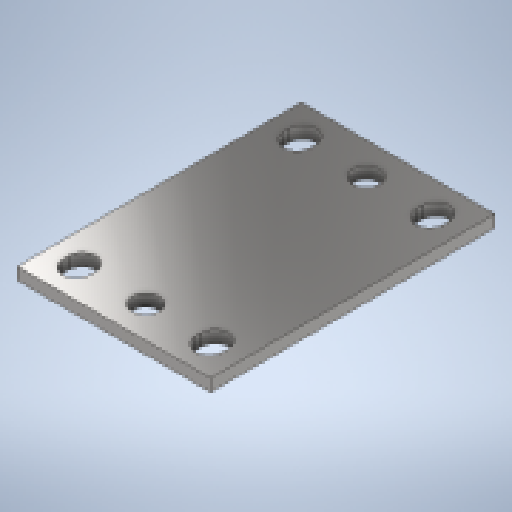
# Autodesk Inventor part: motor_bracket_upper
Saved by Autodesk Inventor 2026.2 (Build 302298010, 298A)
## iProperties
Created: 2026-03-29
Part Number: motor_bracket_upper
Material: Steel, Alloy
Document SubType Name: Modeling
Designer: chanh
Density: 7.73 g/cm^3
Appearance: Semi-Polished
Author: chanh
Autodesk Inventor part; units mm, degrees
ref_plane "YZ Plane" through (0, 0, 0) normal (1, 0, 0) x (0, 1, 0)
ref_plane "XZ Plane" through (0, 0, 0) normal (0, 1, 0) x (-1, 0, 0)
ref_plane "XY Plane" through (0, 0, 0) normal (0, 0, 1) x (1, 0, 0)
sketch "Sketch1" plane through (0, 0, 0) normal (0, 1, 0) x (-1, 0, 0)
  circle A0 centre (0, 0) radius 20
  dimension "d0" = 40
  constraints: 1 centre point, 1 coincident
  measures "d0" diameter of A0
extrude "Extrusion1" add sketch "Sketch1" along normal blind 5
sketch "Sketch2" plane through (0, 5, 0) normal (0, 1, 0) x (1, 0, 0)
  line L0 (-32, -47) -> (32, -47)
  line L1 (32, -47) -> (32, 47)
  line L2 (32, 47) -> (-32, 47)
  line L3 (-32, 47) -> (-32, -47)
  line L4 (-32, -47) -> (32, 47) construction
  line L5 (32, -47) -> (-32, 47) construction
  line L6 (-22, -36.5) -> (22, -36.5) construction
  line L7 (22, -36.5) -> (22, 36.5) construction
  line L8 (22, 36.5) -> (-22, 36.5) construction
  line L9 (-22, 36.5) -> (-22, -36.5) construction
  line L10 (-22, -36.5) -> (22, 36.5) construction
  line L11 (22, -36.5) -> (-22, 36.5) construction
  line L12 (-22, 35.5) -> (-22, 37.5) construction
  line L13 (-17.5, 35.5) -> (-17.5, 37.5)
  line L14 (-26.5, 37.5) -> (-26.5, 35.5)
  arc A0 (-26.5, 35.5) -> (-17.5, 35.5) centre (-22, 35.5) ccw
  arc A1 (-17.5, 37.5) -> (-26.5, 37.5) centre (-22, 37.5) ccw
  line L15 (-32, 0) -> (32, 0) construction
  line L16 (0, 47) -> (0, -47) construction
  line L17 (17.5, 35.5) -> (17.5, 37.5)
  line L18 (26.5, 37.5) -> (26.5, 35.5)
  arc A2 (17.5, 35.5) -> (26.5, 35.5) centre (22, 35.5) ccw
  arc A3 (26.5, 37.5) -> (17.5, 37.5) centre (22, 37.5) ccw
  line L19 (-17.5, -35.5) -> (-17.5, -37.5)
  line L20 (-26.5, -37.5) -> (-26.5, -35.5)
  arc A4 (-17.5, -35.5) -> (-26.5, -35.5) centre (-22, -35.5) ccw
  arc A5 (-26.5, -37.5) -> (-17.5, -37.5) centre (-22, -37.5) ccw
  arc A6 (17.5, -37.5) -> (26.5, -37.5) centre (22, -37.5) ccw
  line L21 (26.5, -37.5) -> (26.5, -35.5)
  arc A7 (26.5, -35.5) -> (17.5, -35.5) centre (22, -35.5) ccw
  line L22 (17.5, -35.5) -> (17.5, -37.5)
  circle A8 centre (0, 36.5) radius 4.5
  circle A9 centre (0, -36.5) radius 4.5
  point P0 (0, 0)
  dimension "d3" = 64
  dimension "d4" = 94
  dimension "d5" = 44
  dimension "d6" = 73
  dimension "d7" = 1
  dimension "d8" = 9
  dimension "d9" = 9
  dimension "d10" = 9
  constraints: 48 end point, 18 symmetric about line, 16 point on circle, 11 midpoint, 10 centre point, 5 parallel, 4 tangent, 3 point on line, 2 horizontal, 2 perpendicular, 6 other
  measures "d3" distance of L1.end L2.end
  measures "d4" distance between parallel lines of L2 L0
  measures "d5" distance of L7.end L8.end
  measures "d6" distance of L6.end L7.end
  measures "d7" distance of L8.end L12.end
  measures "d8" diameter of A1
  measures "d9" diameter of A8
  measures "d10" diameter of A9
extrude "Extrusion2" add sketch "Sketch2" along normal blind 4
body "Solid1"
